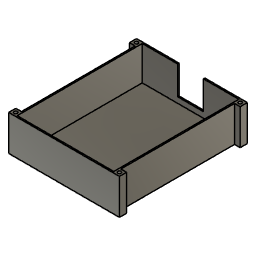
Leserhalter v7 (Autodesk Fusion 360 design; units mm, degrees)
Autodesk Fusion 360 part; units mm, degrees
note: some values were not read from the file. Chosen so that the rebuilt part matches the saved one: which bodies a step acts on; which face or edge a step refers to.
box "Grundkörper Quader1" add length 90 width 70 height 25 placed x (0, 1, 0) y (-1, 0, 0) z (0, 0, 1) at (70, 0, 0) makes body 1
shell "Schale1" thickness 1 removed faces 1 at (23.3333, 30, 25) on bodies 1
fillet "Abrundung1" radius 1 1 edges at (70, 0, 12.5) on bodies 1
fillet "Abrundung2" radius 1 1 edges at (0, 0, 12.5) on bodies 1
fillet "Abrundung3" radius 1 1 edges at (0, 90, 12.5) on bodies 1
fillet "Abrundung4" radius 1 1 edges at (70, 90, 12.5) on bodies 1
box "Grundkörper Quader2" add length 5 width 5 height 25 placed x (0, 1, 0) y (-1, 0, 0) z (0, 0, 1) at (109.8348, 7.8724, 1) separate body makes body 2
hole "Bohrung1" at (107.3348, 10.3724, 26) direction (0, 0, -1) diameter 2.4 depth 25 tip angle 180 bodies 2
copy_body "Körper kopieren/einfügen1" bodies 2 makes body 3
move_body "Verschieben1" bodies 3 to x (1, 0, 0) y (0, 1, 0) z (0, 0, 1) at (-19.3445, -12.5667, 13.2356)
move_body "Verschieben2" bodies 3 to x (1, 0, 0) y (0, 1, 0) z (0, 0, 1) at (-12.7641, -5.6652, -8.6537)
move_body "Verschieben3" bodies 3 to x (1, 0, 0) y (0, 1, 0) z (0, 0, 1) at (1, 0, 0)
move_body "Verschieben4" bodies 3 to x (1, 0, 0) y (0, 1, 0) z (0, 0, 1) at (-4.7261, 10.3595, -5.582)
copy_body "Körper kopieren/einfügen2" bodies 3 makes body 4
copy_body "Körper kopieren/einfügen3" bodies 3 makes body 5
move_body "Verschieben5" bodies 5 to x (1, 0, 0) y (0, 1, 0) z (0, 0, 1) at (-100.0491, 0, -0.5182)
move_body "Verschieben6" bodies 5 to x (1, 0, 0) y (0, 1, 0) z (0, 0, 1) at (27.0491, 0, 0.5182)
move_body "Verschieben7" bodies 2 to x (1, 0, 0) y (0, 1, 0) z (0, 0, 1) at (-35.8348, 77.1276, -1)
move_body "Verschieben8" bodies 4 to x (1, 0, 0) y (0, 1, 0) z (0, 0, 1) at (-97.7252, 90.0766, 0.3044)
move_body "Verschieben9" bodies 4 to x (1, 0, 0) y (0, 1, 0) z (0, 0, 1) at (24.7252, -5.0766, -0.3044)
combine "Kombinieren1" operation add target body 1 tool bodies 2 3 4 5
box "Grundkörper Quader3" add length 30 width 18 height 30 placed x (0, 1, 0) y (-1, 0, 0) z (0, 0, 1) at (44.6699, 119.0681, 0) separate body makes body 6
move_body "Verschieben10" bodies 6 to x (1, 0, 0) y (0, 1, 0) z (0, 0, 1) at (0, -30, 0)
move_body "Verschieben11" bodies 6 to x (1, 0, 0) y (0, 1, 0) z (0, 0, 1) at (5, 0, 0)
move_body "Verschieben12" bodies 6 to x (1, 0, 0) y (0, 1, 0) z (0, 0, 1) at (24.3301, 0.9319, 0)
move_body "Verschieben13" bodies 6 to x (1, 0, 0) y (0, 1, 0) z (0, 0, 1) at (-30, 0, 0)
move_body "Verschieben14" bodies 6 to x (1, 0, 0) y (0, 1, 0) z (0, 0, 1) at (0, 5, 0)
move_body "Verschieben15" bodies 6 to x (1, 0, 0) y (0, 1, 0) z (0, 0, 1) at (0, -10, 0)
move_body "Verschieben16" bodies 6 to x (1, 0, 0) y (0, 1, 0) z (0, 0, 1) at (0, 0, 5)
split "Teilen1" by bodies 6 bodies 1 makes body 7 at (46.6667, 58.3333, 0)
hidden bodies 1 6
named bodies: "Grundkörper", "Schraube1", "Schraube2", "Schraube4", "Schraube3", "Grundkörper (1)"
